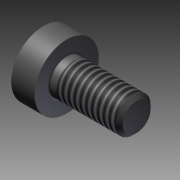
# Autodesk Inventor part: CBSH3-6
Saved by Autodesk Inventor 2011 SP1 (Build 150282100, 282)
## iProperties
Created: 2016-04-08
Part Number: CBSH3-6
Catalog Web Link: www.cadenas.de
Description: CBSH, CBSSTH-Hexagon Socket Extra Low Head Cap Screws High Strength Type
Vendor: MISUMI
Document SubType Name: Modeling
Designer: psAdmin
Manufacturer: MISUMI
Mass: 0.0840593 g
Surface Area: 1.46911 cm^2
Volume: 0.0840593 cm^3
Density: 1 g/cm^3
Category: PARTsolutions
Company: MISUMI
Title: CBSH3-6
Author: Cadenas PARTsolutions
Comments: Hexagon Socket Extra Low Head Cap Screws High Strength Type
PSOL_IDENT_0: {$CADENAS_DATA\23d-libs\misumi\metric\27_screws_nuts\cbsh.prj},167 {VTYP=3D},{NB=CBSH3-6},{LINA=CBSH
PSOL_IDENT_1: 3-6},{NN=CBSH, CBSSTH},{DATE=29.07.2015 04:50:04},{GEOMDATE=27.02.2012 00:00:00},{VERSION=},{LINEID=
PSOL_IDENT_2: 10},{LINESUBID=-1},{WBVAR=MAT,L}  {NB=CBSH3-6},{LINA=CBSH3-6},{KT=DUMMY},{PN=CBSH3-6},{TYPE=CBSH},{M
PSOL_IDENT_3: AT=},{MAT0= '','4137 Alloy Steel','ST','316L Stainless Steel' },{HARD=32~39HRC},{ST=Black Oxide},{SC=
PSOL_IDENT_4: 10.9},{M=3},{L=6},{LALG=4,5,6,8,10,12},{LL=Full Thread},{L0=4,5,6,8,10,12},{L1=4,5,6,8,10},{MP=3x0.5
PSOL_IDENT_5: },{PITCH=0.50},{A=5.5},{E=2.0},{B=2.0},{TT=1.5},{RR=0.1 or More},{RR0=0.10}
NN: CBSH, CBSSTH
NT: Hexagon Socket Extra Low Head Cap Screws High Strength Type
NB: CBSH3-6
NBSYN: $PN.
LINA: CBSH3-6
PN: CBSH3-6
MAT: 4137 Alloy Steel
HARD: 32~39HRC
ST: Black Oxide
SC: 10.9
M: 3
L: 6
LL: Full Thread
MP: 3x0.5
A: 5.5
E: 2.0
B: 2.0
TT: 1.5
RR: 0.1 or More
SUPPLIER: MISUMI
ARTICLENO: CBSH3-6
BOMINFO: CBSH3-6
CREATOR: CADENAS GmbH
Autodesk Inventor part; units mm, degrees
ref_plane "YZ Plane" through (0, 0, 0) normal (1, 0, 0) x (0, 1, 0)
ref_plane "XZ Plane" through (0, 0, 0) normal (0, 1, 0) x (-1, 0, 0)
ref_plane "XY Plane" through (0, 0, 0) normal (0, 0, 1) x (1, 0, 0)
sketch "Sketch_1" plane through (0, 0, 0) normal (0, 0, 1) x (1, 0, 0)
  line L0 (6, 0) -> (-0.2321, 0)
  line L1 (-0.2321, 0) -> (-0.5, 1)
  line L2 (-0.5, 1) -> (-2, 1)
  line L3 (-2, 1) -> (-2, 2.75)
  line L4 (-2, 2.75) -> (0, 2.75)
  line L5 (0, 2.75) -> (0, 1.6)
  arc A0 (0, 1.6) -> (0.1, 1.5) centre (0.1, 1.6) ccw
  line L6 (0.1, 1.5) -> (5.6935, 1.5)
  line L7 (5.6935, 1.5) -> (6, 1.1935)
  line L8 (6, 1.1935) -> (6, 0)
  line L9 (6, 0) -> (-0.2321, 0)
  constraints: 20 end point, 2 point on circle, 1 centre point
revolve "Revolution1" add sketch "Sketch_1" angle 360 about axis through (6, 0, 0) along (1, 0, 0)
thread "Thread1" size "M3x0.5" class "6g" standard "ISO Metric profile" length 5.0626
sketch "Sketch_2" plane through (-2, 0, 0) normal (1, 0, 0) x (0, 0, -1)
  line L0 (-1, 0.5774) -> (-1, -0.5774)
  line L1 (-1, -0.5774) -> (0, -1.1547)
  line L2 (0, -1.1547) -> (1, -0.5774)
  line L3 (1, -0.5774) -> (1, 0.5774)
  line L4 (1, 0.5774) -> (0, 1.1547)
  line L5 (0, 1.1547) -> (-1, 0.5774)
  constraints: 12 end point
extrude "Extrusion1" cut sketch "Sketch_2" along normal blind 1.5
body "Solid1"
